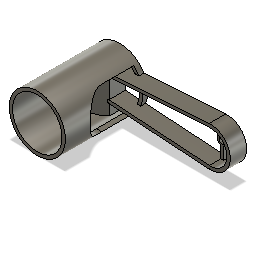
sg90-bucket-and-rail (Autodesk Fusion 360 design; units mm, degrees)
Autodesk Fusion 360 part; units mm, degrees
sketch "Sketch1" plane through (0, 0, 0) normal (0, 0, 1) x (1, 0, 0)
  line L0 (-75, 0) -> (0, 0) construction
  line L1 (-75.3333, -4.9889) -> (-0.6667, -9.9778)
  arc A0 (-0.6667, -9.9778) -> (-0.6667, 9.9778) centre (0, 0) ccw
  line L2 (-0.6667, 9.9778) -> (-75.3333, 4.9889)
  arc A1 (-75.3333, 4.9889) -> (-75.3333, -4.9889) centre (-75, 0) ccw
  circle A2 centre (-65, 0) radius 15
  circle A3 centre (-61.5, 0) radius 11.5 construction
  line L3 (1, -9.9499) -> (1, 9.9499)
  line L4 (-1, -9.9555) -> (-1, 9.9555)
  circle A4 centre (0, 0) radius 3
  circle A5 centre (0, 0) radius 0.8
  line L5 (-74, -5.078) -> (-74, 5.078)
  line L6 (-76, -4.899) -> (-76, 4.899)
  circle A6 centre (-75, 0) radius 3
  circle A7 centre (-75, 0) radius 0.8
  line L7 (-61.5, -14.586) -> (-61.5, 14.586)
  circle A8 centre (-65, 0) radius 17
  line L8 (-0.8, 11.9733) -> (-75.4667, 6.9844)
  arc A9 (-75.4667, 6.9844) -> (-75.4667, -6.9844) centre (-75, 0) ccw
  line L9 (-75.4667, -6.9844) -> (-0.8, -11.9733)
  arc A10 (-0.8, -11.9733) -> (-0.8, 11.9733) centre (0, 0) ccw
  circle A11 centre (-75, 0) radius 5
  point P0 (-80, 0)
  point P1 (-73, 0)
  point P2 (-50, 0)
  point P3 (-50, 0)
  dimension "d1" = 75
  dimension "d2" = 10
  dimension "d3" = 5
  dimension "d4" = 30
  dimension "d5" = 23
  dimension "d6" = 2
  dimension "d7" = 2
  dimension "d8" = 1
  dimension "d9" = 1
  dimension "d10" = 6
  dimension "d11" = 1.6
  dimension "d12" = 1
  dimension "d13" = 1
  dimension "d14" = 6
  dimension "d15" = 1.6
  dimension "d34" = 2
  constraint coincident L0.end A0.centre
  constraint horizontal L0
  constraint tangent L1 A0
  constraint tangent A0 L2
  constraint tangent L2 A1
  constraint tangent L1 A1
  constraint coincident L0.start A1.centre
  constraint coincident A2 P0
  constraint midpoint A1 P0
  constraint coincident L0 A2.centre
  constraint coincident A0 L3.end
  constraint vertical L3
  constraint coincident L2 L4.end
  constraint vertical L4
  constraint coincident L1 L5.start
  constraint vertical L5
  constraint coincident A1 L6.start
  constraint coincident A1 L6.end
  constraint vertical L6
  constraint concentric A6 A9
  constraint concentric A7 A9
  constraint coincident A0 L3.start
  constraint coincident L1 L4.start
  constraint coincident L2 L5.end
  constraint vertical L7
  constraint coincident A3 P1
  constraint coincident A2 L7.end
  constraint coincident A2 L7.start
  constraint coincident A3 P3
  constraint coincident L0 P3
  constraint coincident A2 P3
  constraint coincident P3 P2
  constraint coincident L0 A3.centre
  constraint midpoint A3.centre L7
  measures "d1" horizontal distance of L0.start L0.end
  measures "d2" radius of A0
  measures "d3" radius of A1
  measures "d4" diameter of A2
  measures "d5" diameter of A3
  measures "d8" distance of L4 L0.end
  measures "d9" distance of L3 L0.end
  measures "d10" diameter of A4
  measures "d11" diameter of A5
  measures "d12" distance of L5 L0.start
  measures "d13" distance of L6 L0.start
  measures "d14" diameter of A6
  measures "d15" diameter of A7
sketch "Sketch2" plane through (0, 0, 0) normal (1, 0, 0) x (0, 0, -1)
  line L0 (0, -12.5) -> (0, 12.5)
  line L1 (-11, 5) -> (0, 5) construction
  line L2 (0, 0) -> (-22.4564, 0) construction
  circle A0 centre (-22.4564, 0) radius 12.5
  line L3 (-22.4564, 12.5) -> (0, 12.5)
  line L4 (-22.4564, -12.5) -> (0, -12.5)
  dimension "d16" = 25
  dimension "d17" = 11
  dimension "d19" = 5
  dimension "d20" = 25
  constraint midpoint L2.start L0
  constraint horizontal L1
  constraint coincident L0 L1.end
  constraint perpendicular L0 L1
  constraint coincident L2.start origin
  constraint perpendicular L0 L2
  constraint coincident L2.end A0.centre
  constraint coincident L1.start A0
  constraint coincident A0 L3.start
  constraint tangent A0 L3
  constraint coincident A0 L4.start
  constraint tangent A0 L4
  measures "d16" vertical distance of L0.start L0.end
  measures "d17" horizontal distance of L1.start L1.end
  measures "d19" distance of L2.start L1
  measures "d20" diameter of A0
extrude "Extrude1" add sketch "Sketch1" along normal blind 50 contours A2 A9 | L1 L2 A2 A8 | L1 A2 A8 L9 | A2 A8 L8 A9 | A2 A8 A9 L9 | L2 A2 A8 L8
extrude "Extrude2" cut sketch "Sketch2" against normal blind 70
extrude "Extrude3" add sketch "Sketch1" along normal blind 10 contours L1 A1 A2 L7 A9 L9 A11 | L1 A2 L7 L9 | L2 A1 A2 L7 L8 A9 A11 | L1 A2 A8 L9 | L2 A2 L7 L8 | L1 A0 L2 A8 L8 L9 A10 | L2 A2 A8 L8
extrude "Extrude4" add sketch "Sketch1" along normal blind 3 contours L1 L5 A11 | A1 L5 L6 A6 A11 | L6 A6 | L5 L6 A6 | L5 A6 | L1 L2 A2 A8 | A1 L5 L6 A6 A11 | A2 A8 L8 A9 | A2 A8 A9 L9 | L2 L5 A11 | L1 A0 L3 L4 A4 | L4 A4 | L3 L4 A4 | A0 L2 L3 L4 A4 | L3 A4
chamfer "Chamfer1" distance 1 angle 45 2 edges at (-0.7459, 0.2893, 3) (-75.7459, 0.2893, 3)
extrude "Extrude5" add sketch "Sketch1" along normal blind 20 contours L1 L5 A11 | L1 A1 A2 L7 A9 L9 A11 | A1 L5 L6 A6 A11 | L1 L2 L5 L7 A11 | A1 L6 A6 A11 | L5 A6 A11 | L2 A1 A2 L7 L8 A9 A11 | A2 L7 A9 L9 | A1 L5 L6 A6 A11 | A2 L7 L8 A9 | L2 L5 A11
chamfer "Chamfer2" distance 17.999 angle 30 1 edges at (-61.5, 0, 20) measured on face at (-65, 0, 20)
shell "Shell1" thickness 2 removed faces 1 at (-70.2264, -7.5276, 0)
extrude "Extrude6" add sketch "Sketch1" along normal blind 2 contours A1 L5 L6 A6 A11 | A1 L6 A6 A11 | L5 A6 A11 | L6 A6 | L5 L6 A6 | L5 A6 | A1 L5 L6 A6 A11
named bodies: "SG90 bucket and rail"
